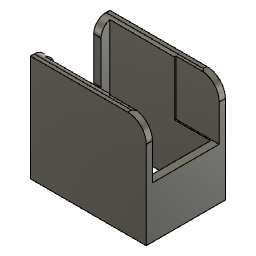
game mounting linear act v8 (Autodesk Fusion 360 archive; units mm, degrees)
design "limitswitch_home"
Autodesk Fusion 360 part; units mm, degrees
sketch "Sketch1" plane through (0, 0, 0) normal (0, 1, 0) x (1, 0, 0)
  line L0 (0, 0) -> (16.3, 0)
  line L1 (16.3, 0) -> (16.3, -10.4)
  line L2 (16.3, -10.4) -> (0, -10.4)
  line L3 (0, -10.4) -> (0, 0)
  line L4 (-1.2, -11.6) -> (-1.2, 1.2)
  line L5 (-1.2, 1.2) -> (17.5, 1.2)
  line L6 (17.5, 1.2) -> (17.5, -11.6)
  line L7 (17.5, -11.6) -> (-1.2, -11.6)
  dimension "d1" = 16.3
  dimension "d2" = 10.4
  dimension "d3" = -1.2
  constraint horizontal L0
  constraint vertical L1
  constraint horizontal L2
  constraint vertical L3
  constraint coincident L0.start L3.end
  measures "d1" distance of L0.start L0.end
  measures "d2" distance of L0.start L2.end
extrude "Extrude1" add sketch "Sketch1" along normal blind 17.2
sketch "Sketch2" plane through (0, 0, 0) normal (1, 0, 0) x (0, 0, -1)
  line L0 (-10.4, 0) -> (0, 0)
  line L1 (0, 0) -> (0, 17.2)
  line L2 (0, 17.2) -> (-10.4, 17.2)
  line L3 (-10.4, 17.2) -> (-10.4, 0)
  line L4 (0, 0) -> (-10.4, 0)
  line L5 (-10.4, 0) -> (-10.4, 0.8)
  line L6 (-10.4, 0.8) -> (0, 0.8)
  line L7 (0, 0.8) -> (0, 0)
  dimension "d6" = 0.8
  constraint horizontal L4
  constraint vertical L5
  constraint horizontal L6
  constraint vertical L7
  constraint coincident L0.end L1.start
  measures "d6" distance of L0.end L6.end
extrude "Extrude2" add sketch "Sketch2" along normal blind 2.3 contours L0 L1 L3 L4 L5 L6 L7
sketch "Sketch3" plane through (16.3, 0, 0) normal (-1, 0, 0) x (0, 0, 1)
  line L0 (0, 0) -> (10.4, 0)
  line L1 (10.4, 0) -> (10.4, 17.2)
  line L2 (10.4, 17.2) -> (0, 17.2)
  line L3 (0, 17.2) -> (0, 0)
  line L4 (10.4, 0) -> (0, 0)
  line L5 (0, 0) -> (0, 0.8)
  line L6 (0, 0.8) -> (10.4, 0.8)
  line L7 (10.4, 0.8) -> (10.4, 0)
  dimension "d9" = 0.8
  constraint horizontal L4
  constraint vertical L5
  constraint horizontal L6
  constraint vertical L7
  constraint coincident L0.end L1.start
  measures "d9" distance of L0.end L6.end
extrude "Extrude3" add sketch "Sketch3" along normal blind 2.2 contours L0 L1 L3 L4 L5 L6 L7
sketch "Sketch4" plane through (17.5, 0, 0) normal (1, 0, 0) x (0, 0, -1)
  line L0 (-11.6, 0) -> (1.2, 0)
  line L1 (1.2, 0) -> (1.2, 17.2)
  line L2 (1.2, 17.2) -> (-11.6, 17.2)
  line L3 (-11.6, 17.2) -> (-11.6, 0)
  line L4 (-5.2, 0) -> (-5.2, 8.3) construction
  line L5 (1.2, 8.3) -> (-11.6, 8.3)
  line L6 (-10.6, 17.2) -> (-10.6, 8.3)
  line L7 (0.2, 17.2) -> (0.2, 8.3)
  dimension "d12" = 8.3
  dimension "d13" = 1
  constraint midpoint L0 L4.start
  constraint perpendicular L0 L4
  constraint coincident L1 L5.start
  constraint coincident L3 L5.end
  constraint perpendicular L3 L5
  constraint coincident L2 L6.start
  constraint coincident L5 L6.end
  constraint perpendicular L5 L6
  constraint symmetric L4 L6.start L7.start
  constraint symmetric L4 L6.end L7.end
  measures "d12" distance of L4.start L4.end
  measures "d13" distance of L3 L6
extrude "Extrude4" cut sketch "Sketch4" against normal blind 7 contours L2 L5 L6 L7
fillet "Fillet1" radius 3 2 edges at (17.5, 17.2, 11.1) (17.5, 17.2, -0.7)
sketch "Sketch5" plane through (-1.2, 0, 0) normal (-1, 0, 0) x (0, 0, 1)
  line L0 (-1.2, 0) -> (11.6, 0)
  line L1 (11.6, 0) -> (11.6, 17.2)
  line L2 (11.6, 17.2) -> (-1.2, 17.2)
  line L3 (-1.2, 17.2) -> (-1.2, 0)
  line L4 (-1.2, 8.3) -> (11.6, 8.3) construction
  line L5 (5.2, 17.2) -> (5.2, 8.3)
  line L6 (1.4, 17.2) -> (1.4, 8.3)
  line L7 (9, 17.2) -> (9, 8.3)
  line L8 (1.4, 8.3) -> (9, 8.3)
  dimension "d18" = 8.3
  dimension "d19" = 2.6
  constraint coincident L3 L4.start
  constraint coincident L1 L4.end
  constraint perpendicular L1 L4
  constraint midpoint L2 L5.start
  constraint midpoint L4 L5.end
  constraint coincident L2 L6.start
  constraint coincident L4 L6.end
  constraint perpendicular L4 L6
  constraint symmetric L5 L6.start L7.start
  constraint symmetric L5 L6.end L7.end
  measures "d18" distance of L0 L4
  measures "d19" distance of L3 L6
extrude "Extrude5" cut sketch "Sketch5" against normal blind 4 contours L2 L5 L6 L8 | L2 L5 L7 L8
fillet "Fillet2" radius 2 2 edges at (-0.6, 17.2, 1.4) (-0.6, 17.2, 9)
equation "d1 = 15.8 mm + 0.5 mm"
equation "d2 = 9.9 mm + 0.5 mm"
